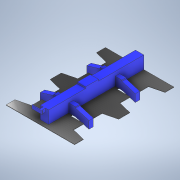
# Autodesk Inventor part: chassis
Saved by Autodesk Inventor 2021 (Build 250183000, 183)
## iProperties
Created: 2020-11-19
Part Number: chassis
Material: Generic
Document SubType Name: Modeling
Designer: Mateusz
Density: 1 g/cm^3
Appearance: Default
Author: Mateusz
Autodesk Inventor part; units mm, degrees
ref_plane "YZ Plane" through (0, 0, 0) normal (1, 0, 0) x (0, 1, 0)
ref_plane "XZ Plane" through (0, 0, 0) normal (0, 1, 0) x (-1, 0, 0)
ref_plane "XY Plane" through (0, 0, 0) normal (0, 0, 1) x (1, 0, 0)
ref_plane "Work Plane1" through (-479.9998, 3, -645.0001) normal (0, 1, 0) x (1, 0, 0)
sketch "Sketch1" plane through (-479.9998, 3, -645.0001) normal (0, 1, 0) x (1, 0, 0)
  line L0 (-140.0002, -474.9989) -> (-260.0002, -474.9989)
  line L1 (-260.0002, -474.9989) -> (-260.0002, -514.9996)
  line L2 (-260.0002, -514.9996) -> (-380.0002, -544.9996)
  line L3 (-380.0002, -544.9996) -> (-380.0002, -625.0004)
  line L4 (-380.0002, -625.0004) -> (240.0001, -625.0004)
  line L5 (240.0001, -625.0004) -> (240.0001, -545.0003)
  line L6 (240.0001, -545.0003) -> (120.0001, -515.0003)
  line L7 (120.0001, -515.0003) -> (120.0001, -474.9989)
  line L8 (120.0001, -474.9989) -> (0, -474.9989)
  line L9 (0, -474.9989) -> (0.0003, -419.9989)
  line L10 (0.0003, -419.9989) -> (0.0003, -349.9996)
  line L11 (0.0003, -349.9996) -> (-0.0003, -295.0009)
  line L12 (-0.0003, -295.0009) -> (120.0001, -294.9996)
  line L13 (120.0001, -294.9996) -> (120.0001, -255.0003)
  line L14 (120.0001, -255.0003) -> (240, -225)
  line L15 (240, -225) -> (240, -125)
  line L16 (240, -125) -> (120, -95)
  line L17 (120, -95) -> (120, 0)
  line L18 (120, 0) -> (0, 0)
  line L19 (0, 0) -> (0, 70)
  line L20 (0, 70) -> (120, 70)
  line L21 (120, 70) -> (120, 165)
  line L22 (120, 165) -> (240, 195)
  line L23 (240, 195) -> (240, 274.9997)
  line L24 (240, 274.9997) -> (-380.0002, 274.9997)
  line L25 (-380.0002, 274.9997) -> (-380.0002, 194.9997)
  line L26 (-380.0002, 194.9997) -> (-260.0002, 164.9996)
  line L27 (-260.0002, 164.9996) -> (-260.0002, 99.9996)
  line L28 (-260.0002, 99.9996) -> (-260.0002, 70)
  line L29 (-260.0002, 70) -> (-140.0002, 70)
  line L30 (-140.0002, 70) -> (-140.0002, 0)
  line L31 (-140.0002, 0) -> (-260.0002, 0)
  line L32 (-260.0002, 0) -> (-260.0002, -30)
  line L33 (-260.0002, -30) -> (-260.0002, -94.9996)
  line L34 (-260.0002, -94.9996) -> (-380.0002, -124.9996)
  line L35 (-380.0002, -124.9996) -> (-380.0002, -224.9996)
  line L36 (-380.0002, -224.9996) -> (-260.0002, -254.9996)
  line L37 (-260.0002, -254.9996) -> (-260.0002, -294.9996)
  line L38 (-260.0002, -294.9996) -> (-140.0002, -294.9996)
  line L39 (-140.0002, -294.9996) -> (-140.0002, -474.9989)
extrude "Extrusion1" add sketch "Sketch1" along normal blind 3
sketch "Sketch2" plane through (-479.9998, 6, -645.0001) normal (0, 1, 0) x (1, 0, 0)
  line L0 (240, 274.9997) -> (-380.0002, 274.9997) projected
  line L1 (-70.0001, -588.0003) -> (-107.7001, -588.0003)
  line L2 (-107.7001, -588.0003) -> (-32.3001, -588.0003)
  line L3 (-32.3001, -588.0003) -> (-32.3001, 274.9997)
  line L4 (-107.7001, -588.0003) -> (-107.7001, 274.9997)
  line L5 (-32.3001, 274.9997) -> (-107.7001, 274.9997)
  point P0 (479.9998, -645.0001)
  dimension "d4" = 37.7
  dimension "d5" = 75.4
  constraints: 10 end point, 3 point on line, 2 perpendicular, 1 collinear, 1 horizontal
  measures "d4" distance of L1.start L1.end
  measures "d5" distance of L1.end L2.end
extrude "Extrusion2" add sketch "Sketch2" along normal blind 115.4
sketch "Sketch3" plane through (-479.9998, 6, -645.0001) normal (0, 1, 0) x (1, 0, 0)
  line L0 (-140.0002, -404.9993) -> (-107.7001, -404.9993)
  line L1 (-107.7001, -588.0003) -> (-107.7001, 274.9997) projected
  line L2 (-140.0002, -364.9993) -> (0.0003, -364.9993)
  line L3 (0.0003, -404.9993) -> (-107.7001, -404.9993)
  line L4 (0, 15) -> (-140.0002, 15)
  line L5 (-140.0002, 55) -> (0, 55)
  line L6 (-70, -364.9993) -> (28.5, -364.9993)
  line L7 (28.5, -364.9993) -> (-168.5, -364.9993)
  line L8 (-168.5, -364.9993) -> (-168.5, -404.9993)
  line L9 (-168.5, -404.9993) -> (-140.0002, -404.9993)
  line L10 (0.0003, -404.9993) -> (28.5, -404.9993)
  line L11 (28.5, -404.9993) -> (28.5, -364.9993)
  line L12 (0, 55) -> (28.5, 55)
  line L13 (28.5, 55) -> (28.5, 15)
  line L14 (28.5, 15) -> (0, 15)
  line L15 (0, 0) -> (0, 70) projected
  line L16 (-140.0002, 55) -> (-168.5, 55)
  line L17 (-168.5, 55) -> (-168.5, 15)
  line L18 (-168.5, 15) -> (-140.0002, 15)
  point P0 (479.9998, -645.0001)
  dimension "d12" = 40
  dimension "d19" = 98.5
  dimension "d20" = 197
  constraints: 34 end point, 7 point on line, 6 perpendicular, 1 collinear, 1 horizontal, 1 midpoint, 1 parallel
  measures "d12" distance of L4.end L5.start
  measures "d19" distance of L6.start L6.end
  measures "d20" distance of L6.end L7.end
extrude "Extrusion3" add sketch "Sketch3" along normal blind 78.5
sketch "Sketch4" plane through (-479.9998, 6, -645.0001) normal (0, 1, 0) x (1, 0, 0)
  line L0 (0.0003, -404.9993) -> (0.0003, -364.9993) projected
  line L1 (0.0003, -384.9993) -> (0.0003, -349.9993)
  line L2 (0.0003, -349.9993) -> (0.0003, -419.9993)
  line L3 (0, -474.9989) -> (0.0003, -419.9989) projected
  line L4 (0.0003, -419.9993) -> (120.0001, -419.9993)
  line L5 (120.0001, -474.9989) -> (0, -474.9989) projected
  line L6 (120.0001, -419.9993) -> (120.0001, -474.9989)
  line L7 (120.0001, -474.9989) -> (0, -474.9989)
  line L8 (0, -474.9989) -> (0.0003, -419.9993)
  line L9 (0.0003, -419.9989) -> (0.0003, -349.9996) projected
  line L10 (0.0003, -349.9996) -> (-0.0003, -295.0009) projected
  line L11 (0.0003, -349.9996) -> (-0.0003, -295.0009)
  line L12 (-0.0003, -295.0009) -> (120.0001, -294.9996) projected
  line L13 (-0.0003, -295.0009) -> (120.0001, -294.9996)
  line L14 (120.0001, -294.9996) -> (120.0001, -349.9996)
  line L15 (120.0001, -349.9996) -> (0.0003, -349.9996)
  line L16 (-140.0002, -364.9993) -> (-140.0002, -404.9993) projected
  line L17 (-140.0002, -384.9993) -> (-140.0002, -349.9996)
  line L18 (-140.0002, -294.9996) -> (-140.0002, -474.9989) projected
  line L19 (-140.0002, -384.9993) -> (-140.0002, -419.9993)
  line L20 (-140.0002, -294.9996) -> (-140.0002, -474.9989) projected
  arc A0 (-140.0002, -419.9993) -> (-140.0002, -419.9993) centre (-140.0002, 50751.7356) ccw
  line L21 (-140.0002, -419.9993) -> (-140.0002, -474.9989)
  line L22 (-140.0002, -474.9989) -> (-260.0002, -474.9989) projected
  line L23 (-260.0002, -474.9989) -> (-260.0002, -514.9996) projected
  line L24 (-140.0002, -474.9989) -> (-260.0002, -474.9989)
  line L25 (-260.0002, -474.9989) -> (-260.0002, -419.9993)
  line L26 (-260.0002, -419.9993) -> (-140.0002, -419.9993)
  line L27 (-140.0002, -349.9996) -> (-140.0002, -294.9996)
  line L28 (-260.0002, -294.9996) -> (-140.0002, -294.9996) projected
  line L29 (-140.0002, -294.9996) -> (-260.0002, -294.9996)
  line L30 (-260.0002, -294.9996) -> (-260.0002, -349.9996)
  line L31 (-260.0002, -349.9996) -> (-140.0002, -349.9996)
  point P0 (479.9998, -645.0001)
  dimension "d15" = 35
  dimension "d16" = 70
  constraints: 40 end point, 9 point on line, 7 perpendicular, 5 collinear, 2 midpoint, 2 point on circle, 1 centre point, 1 horizontal
  measures "d15" distance of L1.start L1.end
  measures "d16" distance of L1.end L2.end
extrude "Extrusion4" add sketch "Sketch4" against normal up to surface (3 mm away) contours L3 L4 L6 L5 | L10 L12 L14 L15 | L18 L31 L30 L28 | L18 L22 L25 L26
sketch "Sketch5" plane through (-479.9995, 6, -240.0008) normal (0, 0, 1) x (1, 0, 0)
  line L0 (0, 0) -> (28.4997, 0) projected
  line L1 (28.4997, 78.5) -> (-32.3004, 78.5) projected
  line L2 (28.4997, 78.5) -> (28.4997, 68.5)
  line L3 (28.4997, 0) -> (28.4997, 78.5) projected
  line L4 (28.4997, 68.5) -> (150.0967, 31.842)
  line L5 (28.4997, 0) -> (150.0967, -36.658)
  line L6 (150.0967, -36.658) -> (150.0967, 31.842)
  line L7 (28.4997, 68.5) -> (28.4997, 0)
  line L8 (-107.7004, 115.4) -> (-32.3004, 115.4) projected
  line L9 (-70.0004, 115.4) -> (-70.0004, 84.9385)
  line L10 (-140.0008, 0) -> (-168.5005, 0)
  line L11 (-168.5005, 78.5) -> (-107.7004, 78.5)
  line L12 (-168.5005, 78.5) -> (-168.5005, 68.5)
  line L13 (-168.5005, 0) -> (-168.5005, 78.5)
  line L14 (-168.5005, 68.5) -> (-290.0975, 31.842)
  line L15 (-168.5005, 0) -> (-290.0975, -36.658)
  line L16 (-290.0975, -36.658) -> (-290.0975, 31.842)
  line L17 (-168.5005, 68.5) -> (-168.5005, 0)
  point P0 (479.9995, -6)
  dimension "d24" = 10
  constraints: 28 end point, 7 symmetric about line, 2 point on line, 2 vertical, 1 collinear, 1 midpoint, 1 parallel
  measures "d24" distance of L1.start L2.end
extrude "Extrusion5" add sketch "Sketch5" against normal up to surface (40 mm away)
sketch "Sketch6" plane through (-479.9998, 6, -660.0001) normal (0, 0, 1) x (1, 0, 0)
  line L0 (-32.3001, 0) -> (-32.3001, 78.5) projected
  line L1 (0.0003, 0) -> (-32.3001, 0) projected
  line L2 (0.0003, 0) -> (28.5, 0) projected
  line L3 (28.5, 0) -> (150.097, -36.658) projected
  line L4 (150.097, -36.658) -> (150.097, 31.842) projected
  line L5 (150.097, 31.842) -> (28.5, 68.5) projected
  line L6 (28.5, 68.5) -> (28.5, 78.5) projected
  line L7 (-32.3001, 78.5) -> (28.5, 78.5) projected
  line L8 (-290.0972, -36.658) -> (-168.5002, 0) projected
  line L9 (-168.5002, 0) -> (-168.5002, 68.5) projected
  line L10 (-168.5002, 68.5) -> (-290.0972, 31.842) projected
  line L11 (-290.0972, 31.842) -> (-290.0972, -36.658) projected
  point P0 (479.9998, -6)
extrude "Extrusion6" add sketch "Sketch6" against normal up to surface (40 mm away)
sketch "Sketch8" plane through (-479.9998, 121.4, -645.0001) normal (0, 1, 0) x (1, 0, 0)
  line L0 (240, -225) -> (240, -125) projected
  line L1 (240, -175) -> (-32.3001, -174.9996)
  line L2 (-32.3001, 15) -> (-32.3001, -364.9993) projected
  line L3 (-32.3001, -174.9996) -> (-107.7001, -174.9996)
  line L4 (-107.7001, -364.9993) -> (-107.7001, 15) projected
  circle A0 centre (-70.0001, -174.9996) radius 14.9657
  line L5 (-70.0001, -174.9996) -> (-70.0001, -224.9996)
  circle A1 centre (-70.0001, -224.9996) radius 8.3807
  line L6 (-107.7001, 274.9997) -> (-107.7001, -588.0003) projected
  line L7 (-32.3001, -588.0003) -> (-32.3001, 274.9997) projected
  line L8 (-107.7001, -253.6114) -> (-32.3001, -253.6114)
  line L9 (-32.3001, -253.6114) -> (-32.3001, -135.5582)
  line L10 (-32.3001, -135.5582) -> (-107.7001, -135.5582)
  line L11 (-107.7001, -135.5582) -> (-107.7001, -253.6114)
  point P0 (479.9998, -645.0001)
  point P1 (-32.3001, -135.5582)
  point P2 (-107.7001, -135.5582)
  point P3 (-107.7001, -253.6114)
  point P4 (-32.3001, -253.6114)
  dimension "d30" = 50
  constraints: 14 end point, 4 midpoint, 2 centre point, 2 parallel, 2 point on line, 1 coincident, 1 horizontal, 1 perpendicular, 1 vertical
  measures "d30" distance of L5.start L5.end
extrude "Extrusion7" add sketch "Sketch8" along normal blind 13.941 contours L2 L3 A0 L4 L10 | L2 L8 L4 L3 A0 | A0 L5 L3 | L3 A0 | L5 A0 L3 | A1
sketch "Sketch9" plane through (-587.6999, 6, -56.9998) normal (0, 0, 1) x (1, 0, 0)
  line L0 (0, 115.4) -> (75.4, 115.4) projected
  line L1 (37.7, 85.538) -> (47.7, 85.538)
  line L2 (47.7, 85.538) -> (37.7, 85.538)
  line L3 (37.7, 85.538) -> (27.7, 85.538)
  line L4 (27.7, 85.538) -> (27.7, 115.4)
  line L5 (47.7, 85.538) -> (47.7, 115.4)
  line L6 (47.7, 115.4) -> (27.7, 115.4)
  point P0 (587.6999, -6)
  constraints: 12 end point, 3 perpendicular, 3 point on line, 1 collinear, 1 horizontal
extrude "Extrusion8" add sketch "Sketch9" along normal blind 30
sketch "Sketch10" plane through (-587.6999, 6, -26.9998) normal (0, 0, 1) x (1, 0, 0)
  line L0 (47.7, 115.4) -> (27.7, 115.4) projected
  line L1 (47.7, 115.4) -> (53.2, 115.4)
  line L2 (47.7, 115.4) -> (75.4, 115.4) projected
  line L3 (53.2, 115.4) -> (53.2, 85.538)
  line L4 (53.2, 85.538) -> (-40.3, 85.538)
  line L5 (-40.3, 85.538) -> (-40.3, 115.4)
  line L6 (-40.3, 115.4) -> (47.7, 115.4)
  point P0 (587.6999, -6)
  dimension "d39" = 5.5
  dimension "d40" = 93.5
  constraints: 10 end point, 2 perpendicular, 1 collinear, 1 horizontal, 1 point on line
  measures "d39" distance of L0.start L1.end
  measures "d40" distance of L3.end L4.end
extrude "Extrusion9" add sketch "Sketch10" along normal blind 7
body "Solid2"
